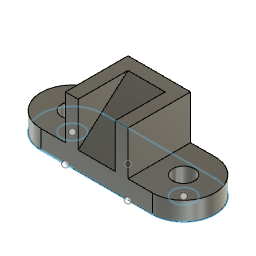
a2 (Autodesk Fusion 360 design; units mm, degrees)
Autodesk Fusion 360 part; units mm, degrees
sketch "Sketch1" plane through (0, 0, 0) normal (0, 0, 1) x (1, 0, 0)
  line L0 (57, 32) -> (-57, 32)
  line L1 (-57, -32) -> (57, -32)
  circle A0 centre (57, 0) radius 11
  circle A1 centre (-57, 0) radius 11
  arc A2 (57, -32) -> (57, 32) centre (57, 0) ccw
  arc A3 (-57, 32) -> (-57, -32) centre (-57, 0) ccw
  line L2 (-57, -32) -> (-32, -32) construction
  line L3 (57, -32) -> (32, -32) construction
  dimension "d1" = 114
  dimension "d2" = 64
  dimension "d3" = 64
  dimension "d4" = 64
  dimension "d5" = 22
  dimension "d6" = 22
  dimension "d9" = 25
  dimension "d10" = 25
  constraint parallel L0 L1
  constraint horizontal L0
  constraint concentric A0 A2
  constraint concentric A1 A3
  constraint parallel L1 L2
  constraint parallel L1 L3
  measures "d1" distance of L1.start L1.end
  measures "d2" distance of L0.end L1.start
  measures "d3" diameter of A2
  measures "d4" diameter of A3
  measures "d5" diameter of A0
  measures "d6" diameter of A1
  measures "d9" distance of L1.start L2.end
  measures "d10" distance of L1.end L3.end
extrude "Extrude1" add sketch "Sketch1" along normal blind 19
sketch "Sketch2" plane through (0, 0, 0) normal (0, 1, 0) x (1, 0, 0)
  line L0 (-32, 0) -> (32, 0)
  line L1 (32, 0) -> (32, -64)
  line L2 (32, -64) -> (-32, -64)
  line L3 (-32, -64) -> (-32, 0)
  dimension "d11" = 64
  constraint horizontal L0
  constraint vertical L1
  constraint horizontal L2
  constraint vertical L3
  measures "d11" distance of L0.start L2.end
extrude "Extrude2" add sketch "Sketch2" along normal mid plane 64
sketch "Sketch3" plane through (0, 0, 64) normal (0, 0, 1) x (-1, 0, 0)
  line L0 (-32, 32) -> (-32, -32)
  line L1 (-32, -32) -> (32, -32)
  line L2 (32, -32) -> (32, 32)
  line L3 (32, 32) -> (-32, 32)
  line L4 (32, 32) -> (32, -19)
  line L5 (-32, 32) -> (-32, -19)
  line L6 (32, 32) -> (19, 32)
  line L7 (-32, 32) -> (-19, 32)
  line L8 (19, 32) -> (19, -19)
  line L9 (-19, 32) -> (-19, -19)
  line L10 (-19, -19) -> (19, -19)
  dimension "d14" = 51
  dimension "d15" = 51
  dimension "d16" = 13
  dimension "d17" = 13
  constraint coincident L2.end L3.start
  constraint perpendicular L3 L4
  constraint coincident L0.start L3.end
  constraint perpendicular L3 L5
  constraint perpendicular L2 L6
  constraint perpendicular L0 L7
  constraint perpendicular L3 L9
  constraint perpendicular L8 L10
  measures "d14" distance of L2.end L4.end
  measures "d15" distance of L0.start L5.end
  measures "d16" distance of L2.end L6.end
  measures "d17" distance of L0.start L7.end
extrude "Extrude3" cut sketch "Sketch3" against normal blind 45 contours L3 L8 L9 L10
sketch "Sketch4" plane through (19, 0, 0) normal (-1, 0, 0) x (0, -1, 0)
  line L0 (32, 64) -> (-19, 64)
  line L1 (-19, 64) -> (-19, 19)
  line L2 (-19, 19) -> (32, 19)
  line L3 (32, 19) -> (32, 64)
  line L4 (-19, 64) -> (32, 19)
  constraint coincident L0.end L1.start
  constraint coincident L2.end L3.start
extrude "Extrude4" add sketch "Sketch4" along normal blind 38 contours L1 L2 L4
